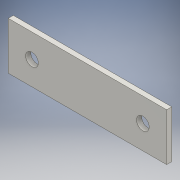
# Autodesk Inventor part: Latch Catch Piece
Saved by Autodesk Inventor 2018 (Build 220112000, 112)
## iProperties
Created: 2018-10-16
Part Number: Latch Catch Piece
Material: Steel
Document SubType Name: Modeling
Designer: P301319
Density: 7.85 g/cm^3
Appearance: Steel
Author: P301319
Autodesk Inventor part; units mm, degrees
ref_plane "YZ Plane" through (0, 0, 0) normal (1, 0, 0) x (0, 1, 0)
ref_plane "XZ Plane" through (0, 0, 0) normal (0, 1, 0) x (-1, 0, 0)
ref_plane "XY Plane" through (0, 0, 0) normal (0, 0, 1) x (1, 0, 0)
sketch "Sketch1" plane through (0, 0, 0) normal (0, 1, 0) x (-1, 0, 0)
  line L0 (0, 0) -> (-50, 0)
  line L1 (-50, 0) -> (-50, -15)
  line L2 (-50, -15) -> (0, -15)
  line L3 (0, -15) -> (0, 0)
  dimension "d0" = 50
  dimension "d1" = 15
  constraints: 8 end point, 2 parallel, 1 horizontal, 1 perpendicular
  measures "d0" distance of L2.end L1.end
  measures "d1" distance of L1.end L0.end
extrude "Extrusion1" add sketch "Sketch1" along normal blind 1.6
sketch "Sketch2" plane through (0, 0, 0) normal (0, -1, 0) x (1, 0, 0)
  circle A0 centre (7.5, -7.5) radius 2
  line L0 (0, -15) -> (0, 0) projected
  circle A1 centre (42.5, -7.5) radius 2
  line L1 (50, 0) -> (50, -15) projected
  point P0 (0, -7.5)
  point P1 (50, -7.5)
  dimension "d4" = 4
  dimension "d5" = 7.5
  dimension "d6" = 4
  dimension "d7" = 7.5
  constraints: 2 centre point, 2 horizontal alignment, 2 midpoint
  measures "d4" diameter of A0
  measures "d5" distance from line of L0 A0.centre
  measures "d6" diameter of A1
  measures "d7" distance from line of L1 A1.centre
extrude "Extrusion2" cut sketch "Sketch2" against normal blind 10
body "Solid1"
